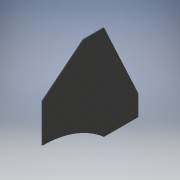
# Autodesk Inventor part: end_plate
Saved by Autodesk Inventor 2018.1 (Build 221171000, 171)
## iProperties
Created: 2017-10-22
Part Number: end_plate
Material: CFRP
Document SubType Name: Modeling
Designer: ku_sk
Density: 1.43 g/cm^3
Appearance: カーボンファイバー
Author: ku_sk
Autodesk Inventor part; units mm, degrees
ref_plane "YZ Plane" through (0, 0, 0) normal (1, 0, 0) x (0, 1, 0)
ref_plane "XZ Plane" through (0, 0, 0) normal (0, 1, 0) x (-1, 0, 0)
ref_plane "XY Plane" through (0, 0, 0) normal (0, 0, 1) x (1, 0, 0)
sketch "スケッチ1" plane through (0, 0, 0) normal (1, 0, 0) x (0, 1, 0)
  line L0 (-700, 170) -> (-700, 450)
  line L1 (-700, 450) -> (-400, 690)
  line L2 (-400, 690) -> (-250, 690)
  line L3 (-250, 690) -> (0, 150)
  line L4 (0, 150) -> (0, 0)
  line L5 (0, 0) -> (-250, 0)
  arc A0 (-250, 0) -> (-700, 170) centre (-700, -510.5882) ccw
  dimension "d0" = 690
  dimension "d1" = 280
  dimension "d2" = 240
  dimension "d3" = 300
  dimension "d4" = 150
  dimension "d5" = 700
  dimension "d6" = 250
  dimension "d7" = 150
  constraints: 12 end point, 2 perpendicular, 2 point on circle, 1 centre point, 1 coincident, 1 horizontal, 1 line through centre, 1 parallel
  measures "d0" distance between parallel lines of L5 L2
  measures "d1" distance of L0.start L0.end
  measures "d2" distance from line of L0.end L2
  measures "d3" distance from line of L1.end L0
  measures "d4" distance of L3.end L4.end
  measures "d5" distance between parallel lines of L0 L4
  measures "d6" distance of L4.end L5.end
  measures "d7" distance of L1.end L2.end
extrude "押し出し1" add sketch "スケッチ1" along normal blind 5
